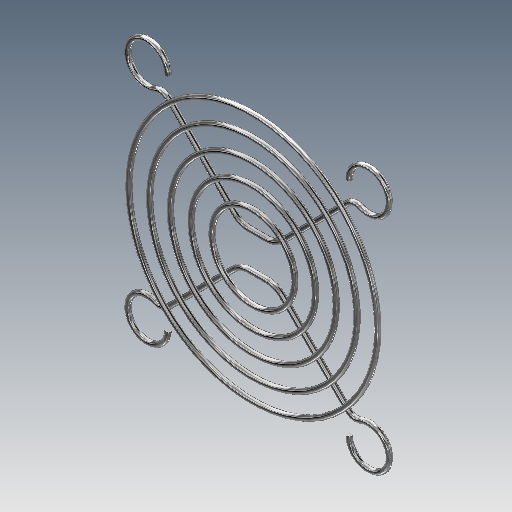
# Autodesk Inventor part: Fan Guard, 40mm
Saved by Autodesk Inventor 2019.1 (Build 231200000, 200)
## iProperties
Created: 2005-12-02
Part Number: Fan Guard, 40mm
Document SubType Name: Modeling
Designer: floress
Density: 1 g/cm^3
Material: Generic
Mass: 0.23414 g
Surface Area: 12.309 cm^2
Volume: 0.23414 cm^3
Appearance: Chrome - Polished
Author: floress
Autodesk Inventor part; units mm, degrees
ref_plane "YZ Plane" through (0, 0, 0) normal (1, 0, 0) x (0, 1, 0)
ref_plane "XZ Plane" through (0, 0, 0) normal (0, 1, 0) x (-1, 0, 0)
ref_plane "XY Plane" through (0, 0, 0) normal (0, 0, 1) x (1, 0, 0)
sketch "Sketch1" plane through (0, 0, 0) normal (0, 0, 1) x (1, 0, 0)
  arc A0 (-13.0846, 16) -> (-14.7976, 13.3441) centre (-16, 16) ccw
  line L0 (-13.0204, 13.0204) -> (-3.5097, 3.5097)
  line L1 (-1.2647, 2.5798) -> (1.2647, 2.5798)
  arc A1 (-3.5097, 3.5097) -> (-1.2647, 2.5798) centre (-1.2647, 5.7548) ccw
  arc A2 (-13.0204, 13.0204) -> (-14.7976, 13.3441) centre (-14.1429, 11.8979) ccw
  arc A3 (14.7976, 13.3441) -> (13.0846, 16) centre (16, 16) ccw
  line L2 (13.0204, 13.0204) -> (3.5097, 3.5097)
  arc A4 (14.7976, 13.3441) -> (13.0204, 13.0204) centre (14.1429, 11.8979) ccw
  arc A5 (1.2647, 2.5798) -> (3.5097, 3.5097) centre (1.2647, 5.7548) ccw
  line L3 (0, 0) -> (0, 12.1391)
  dimension "d0" = 3.175
  dimension "d1" = 3.175
  dimension "d10" = 2.9154
  dimension "d11" = 32
  dimension "d13" = 2.5798
  constraints: 12 point on circle, 8 end point, 6 centre point, 4 tangent, 1 perpendicular, 2 other
  measures "d0" radius of A1
  measures "d1" diameter of A2
  measures "d10" radius of A0
  measures "d11" distance of A3.centre A0.centre
  measures "d13" distance from line of L1 L3.start
ref_plane "Work Plane1" through (-13.0846, 16, 0) normal (0, 1, 0) x (-1, 0, 0)
sketch "Sketch2" plane through (-13.0846, 16, 0) normal (0, 1, 0) x (-1, 0, 0)
  circle A0 centre (0, 0) radius 0.381
  dimension "d2" = 0.762
  constraints: 1 centre point
  measures "d2" diameter of A0
sweep "Sweep1" add profiles "Sketch2" path "Sketch1" path curves A0 A2 L0 A1 L1 A5 L2 A4 A3
sketch "Sketch4" plane through (0, 0, 0) normal (0, 0, 1) x (1, 0, 0)
  line L0 (-1.2647, -2.5798) -> (1.2647, -2.5798)
  arc A0 (3.5097, -3.5097) -> (1.2647, -2.5798) centre (1.2647, -5.7548) ccw
  line L1 (13.0204, -13.0204) -> (3.5097, -3.5097)
  arc A1 (13.0846, -16) -> (14.7976, -13.3441) centre (16, -16) ccw
  arc A2 (13.0204, -13.0204) -> (14.7976, -13.3441) centre (14.1429, -11.8979) ccw
  line L2 (0, 0) -> (0, -10.7959)
  arc A3 (-1.2647, -2.5798) -> (-3.5097, -3.5097) centre (-1.2647, -5.7548) ccw
  line L3 (-13.0204, -13.0204) -> (-3.5097, -3.5097)
  arc A4 (-14.7976, -13.3441) -> (-13.0204, -13.0204) centre (-14.1429, -11.8979) ccw
  arc A5 (-14.7976, -13.3441) -> (-13.0846, -16) centre (-16, -16) ccw
  dimension "d14" = 2.9154
  dimension "d15" = 1.5875
  dimension "d16" = 3.175
  dimension "d17" = 2.5798
  constraints: 12 point on circle, 8 end point, 7 symmetric about line, 6 centre point, 1 perpendicular, 3 other
  measures "d14" radius of A1
  measures "d15" radius of A2
  measures "d16" radius of A0
  measures "d17" distance from line of L2.start L0
ref_plane "Work Plane3" through (13.0846, -16, 0) normal (0, -1, 0) x (1, 0, 0)
sketch "Sketch5" plane through (13.0846, -16, 0) normal (0, -1, 0) x (1, 0, 0)
  circle A0 centre (0, 0) radius 0.381
  dimension "d7" = 0.762
  constraints: 1 centre point
  measures "d7" diameter of A0
sweep "Sweep2" add profiles "Sketch5" path "Sketch4" path curves A1 A2 L1 A0 L0 A3 L3 A4 A5
ref_plane "Work Plane4" through (0, 0, 0.762) normal (0, 0, 1) x (1, 0, 0)
sketch "Sketch6" plane through (0, 0, 0.762) normal (0, 0, 1) x (1, 0, 0)
  circle A0 centre (0, 0) radius 18
  dimension "d18" = 36
  constraints: 1 centre point, 1 coincident
  measures "d18" diameter of A0
sketch "Sketch7" plane through (0, 0, 0.762) normal (0, 0, 1) x (1, 0, 0)
  circle A0 centre (0, 0) radius 15
  dimension "d19" = 30
  constraints: 1 centre point
  measures "d19" diameter of A0
sketch "Sketch8" plane through (0, 0, 0.762) normal (0, 0, 1) x (1, 0, 0)
  circle A0 centre (0, 0) radius 12
  dimension "d20" = 24
  constraints: 1 centre point
  measures "d20" diameter of A0
sketch "Sketch9" plane through (0, 0, 0.762) normal (0, 0, 1) x (1, 0, 0)
  circle A0 centre (0, 0) radius 9
  dimension "d21" = 18
  constraints: 1 centre point
  measures "d21" diameter of A0
sketch "Sketch10" plane through (0, 0, 0.762) normal (0, 0, 1) x (1, 0, 0)
  circle A0 centre (0, 0) radius 6
  dimension "d22" = 12
  constraints: 1 centre point
  measures "d22" diameter of A0
sketch "Sketch11" plane through (0, 0, 0) normal (0, 1, 0) x (-1, 0, 0)
  line L0 (18, 0.762) -> (-18, 0.762) projected
  circle A0 centre (-18, 0.762) radius 0.381
  point P0 (0, 0)
  dimension "d23" = 0.762
  constraints: 1 centre point, 1 coincident
  measures "d23" diameter of A0
sketch "Sketch12" plane through (0, 0, 0) normal (0, 1, 0) x (-1, 0, 0)
  line L0 (15, 0.762) -> (-15, 0.762) projected
  circle A0 centre (-15, 0.762) radius 0.381
  dimension "d24" = 0.762
  constraints: 1 centre point, 1 coincident
  measures "d24" diameter of A0
sketch "Sketch13" plane through (0, 0, 0) normal (0, 1, 0) x (-1, 0, 0)
  line L0 (12, 0.762) -> (-12, 0.762) projected
  circle A0 centre (-12, 0.762) radius 0.381
  dimension "d25" = 0.762
  constraints: 1 centre point, 1 coincident
  measures "d25" diameter of A0
sketch "Sketch14" plane through (0, 0, 0) normal (0, 1, 0) x (-1, 0, 0)
  line L0 (9, 0.762) -> (-9, 0.762) projected
  circle A0 centre (-9, 0.762) radius 0.381
  dimension "d26" = 0.762
  constraints: 1 centre point, 1 coincident
  measures "d26" diameter of A0
sketch "Sketch15" plane through (0, 0, 0) normal (0, 1, 0) x (-1, 0, 0)
  line L0 (6, 0.762) -> (-6, 0.762) projected
  circle A0 centre (-6, 0.762) radius 0.381
  dimension "d27" = 0.762
  constraints: 1 centre point, 1 coincident
  measures "d27" diameter of A0
sweep "Sweep3" add profiles "Sketch11" path "Sketch6"
sweep "Sweep4" add profiles "Sketch12" path "Sketch7"
sweep "Sweep5" add profiles "Sketch13" path "Sketch8"
sweep "Sweep6" add profiles "Sketch14" path "Sketch9"
sweep "Sweep7" add profiles "Sketch15" path "Sketch10"
body "Solid1"
